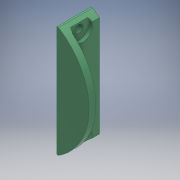
# Autodesk Inventor part: 05-01-Кронштейн низ защита (update)
Saved by Autodesk Inventor 2018 (Build 220112000, 112)
## iProperties
Created: 2018-12-08
Part Number: 05-01-Кронштейн низ защита (update)
Material: Типовые
Document SubType Name: Modeling
Designer: RR
Density: 1 g/cm^3
Appearance: Гладкий — темный цвет морской волны
Author: RR
Autodesk Inventor part; units mm, degrees
ref_plane "YZ Plane" through (0, 0, 0) normal (1, 0, 0) x (0, 1, 0)
ref_plane "XZ Plane" through (0, 0, 0) normal (0, 1, 0) x (-1, 0, 0)
ref_plane "XY Plane" through (0, 0, 0) normal (0, 0, 1) x (1, 0, 0)
sketch "Эскиз1" plane through (0, 0, 0) normal (0, 1, 0) x (-1, 0, 0)
  line L0 (0, -56) -> (0, -121)
  line L1 (0, -56) -> (-1, -56)
  line L2 (0, -56) -> (1, -56) construction
  line L3 (0, -121) -> (-1, -121)
  line L4 (0, -121) -> (1, -121) construction
  arc A0 (-1, -56) -> (-1, -121) centre (19.5, -88.5) ccw
  dimension "d5" = 65
  dimension "d6" = 1
  dimension "d7" = 180
  dimension "d8" = 1
  dimension "d9" = 180
  constraints: 10 end point, 4 horizontal, 2 collinear, 2 point on circle, 1 centre point, 1 vertical
  measures "d5" distance of L0.start L0.end
  measures "d6" distance of L0.start L1.end
  measures "d7" angle of L1 L2
  measures "d8" distance of L0.end L3.end
  measures "d9" angle of L3 L4
extrude "Выдавливание1" add sketch "Эскиз1" along normal blind 4
sketch "Эскиз2" plane through (0, 4, 0) normal (0, 1, 0) x (1, 0, 0)
  line L0 (0, 121) -> (0, 56) projected
  line L1 (0, 56) -> (0, 121)
  line L2 (0, 121) -> (1, 121)
  line L3 (0, 56) -> (1, 56)
  arc A0 (1, 56) -> (1, 121) centre (-19.5, 88.5) ccw projected
  line L4 (5, 58.8985) -> (5, 118.1015)
  arc A1 (1, 56) -> (5, 58.8985) centre (-19.5, 88.5) ccw
  arc A2 (5, 118.1015) -> (1, 121) centre (-19.5, 88.5) ccw
  point P0 (0, 0)
  constraints: 8 end point, 4 point on circle, 2 centre point, 1 collinear, 1 horizontal, 1 perpendicular
extrude "Выдавливание2" add sketch "Эскиз2" along normal blind 16 contours L2 A0 L4 L3 L0
sketch "Эскиз3" plane through (0, 0, -121) normal (-1, 0, 0) x (0, 0, 1)
  line L0 (65, 0) -> (0, 0) projected
  line L1 (32.5, 0) -> (32.5, 20)
  line L2 (0, 20) -> (65, 20) projected
  line L3 (4.5, 10) -> (60.5, 10)
  circle A0 centre (4.5, 10) radius 2.25
  circle A1 centre (60.5, 10) radius 2.25
  point P0 (121, 0)
  dimension "d17" = 4.5
  dimension "d18" = 4.5
  constraints: 4 end point, 2 centre point, 2 coincident, 2 midpoint
  measures "d17" diameter of A0
  measures "d18" diameter of A1
extrude "Выдавливание3" cut sketch "Эскиз3" against normal blind 5
sketch "Эскиз4" plane through (5, 4, -58.8985) normal (1, 0, 0) x (0, 0, -1)
  arc A0 (0, 4.4196) -> (0, 7.5804) centre (1.6015, 6) ccw projected
  circle A1 centre (1.6015, 6) radius 6
  line L0 (59.203, 0) -> (0, 0) projected
  arc A2 (59.203, 7.5804) -> (59.203, 4.4196) centre (57.6015, 6) ccw projected
  circle A3 centre (57.6015, 6) radius 6
  point P0 (-58.8985, -4)
  constraints: 2 centre point, 2 coincident, 1 tangent
extrude "Выдавливание4" cut sketch "Эскиз4" against normal blind 2
